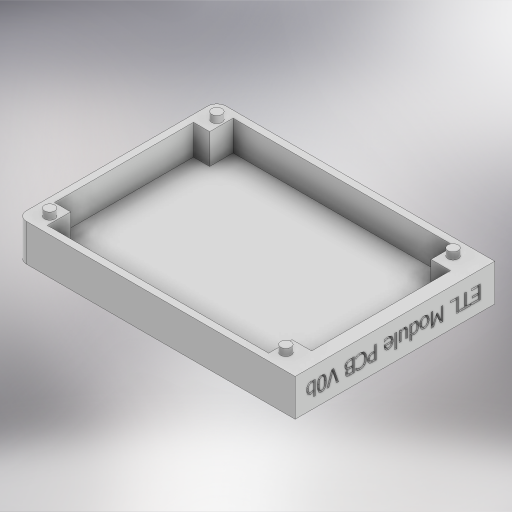
# Autodesk Inventor part: Cover V1
Saved by Autodesk Inventor 2024 (Build 280153000, 153)
## iProperties
Created: 2023-10-11
Part Number: Cover V1
Material: Generic
Document SubType Name: Modeling
Designer: cfang
Density: 1 g/cm^3
Appearance: Default
Author: cfang
Autodesk Inventor part; units mm, degrees
ref_plane "YZ Plane" through (0, 0, 0) normal (1, 0, 0) x (0, 1, 0)
ref_plane "XZ Plane" through (0, 0, 0) normal (0, 1, 0) x (-1, 0, 0)
ref_plane "XY Plane" through (0, 0, 0) normal (0, 0, 1) x (1, 0, 0)
sketch "Sketch1" plane through (0, 0, 0) normal (0, 1, 0) x (-1, 0, 0)
  line L0 (-30, -21.55) -> (30, -21.55)
  line L1 (30, -21.55) -> (30, 21.55)
  line L2 (30, 21.55) -> (-30, 21.55)
  line L3 (-30, 21.55) -> (-30, -21.55)
  line L4 (-30, -21.55) -> (30, 21.55) construction
  line L5 (30, -21.55) -> (-30, 21.55) construction
  point P0 (0, 0)
  dimension "d0" = 43.1
  dimension "d1" = 60
  constraints: 12 end point, 2 midpoint, 2 parallel, 1 horizontal, 1 perpendicular
  measures "d0" distance of L0.end L1.end
  measures "d1" distance of L1.end L2.end
extrude "Extrusion1" add sketch "Sketch1" along normal blind 8
sketch "Sketch2" plane through (0, 8, 0) normal (0, 1, 0) x (1, 0, 0)
  line L0 (22.78, 20.05) -> (-25, 20.05)
  line L1 (-25, 20.05) -> (-25, -20.05)
  line L2 (-25, -20.05) -> (22.78, -20.05)
  line L3 (22.78, -20.05) -> (22.78, 20.05)
  line L4 (-30, -21.55) -> (30, -21.55) projected
  line L5 (30, -21.55) -> (30, 21.55) projected
  line L6 (-30, 21.55) -> (-30, -21.55) projected
  line L7 (30, 21.55) -> (-30, 21.55) projected
  line L8 (22.78, -15) -> (27, -15)
  line L9 (27, -15) -> (27, 15)
  line L10 (27, 15) -> (22.78, 15)
  line L11 (22.78, 15) -> (22.78, -15)
  line L12 (-25, 15) -> (-28.5, 15)
  line L13 (-28.5, 15) -> (-28.5, -15)
  line L14 (-28.5, -15) -> (-25, -15)
  line L15 (-25, -15) -> (-25, 15)
  point P0 (0, 0)
  point P1 (22.78, 15)
  dimension "d4" = 1.5
  dimension "d7" = 7.22
  dimension "d8" = 5
  dimension "d9" = 1.5
  dimension "d24" = 30
  dimension "d25" = 15
  dimension "d26" = 3
  dimension "d27" = 30
  dimension "d28" = 1.5
  dimension "d29" = 15
  constraints: 24 end point, 6 parallel, 3 horizontal, 3 perpendicular, 2 point on line
  measures "d4" distance between parallel lines of L4 L2
  measures "d7" distance between parallel lines of L5 L3
  measures "d8" distance between parallel lines of L6 L1
  measures "d9" distance between parallel lines of L7 L0
  measures "d24" distance of L8.end L9.end
  measures "d25" distance from line of point (0, 0) L10
  measures "d26" distance between parallel lines of L5 L9
  measures "d27" distance of L12.end L13.end
  measures "d28" distance between parallel lines of L6 L13
  measures "d29" distance from line of point (0, 0) L12
extrude "Extrusion2" cut sketch "Sketch2" against normal blind 6.5 contours L3 L2 L1 L0 | L10 L9 L8 L3 | L1 L14 L13 L12
fillet "Fillet1" radius 2 2 edges at (-30, 4, 21.55) (-30, 4, -21.55)
sketch "Sketch3" plane through (0, 8, 0) normal (0, 1, 0) x (1, 0, 0)
  circle A0 centre (24.5, 18.05) radius 1.1
  circle A1 centre (24.5, -18.05) radius 1.1
  line L0 (30, -21.55) -> (30, 21.55) projected
  circle A2 centre (-26.5, 18.05) radius 1.1
  circle A3 centre (-26.5, -18.05) radius 1.1
  line L1 (30, 21.55) -> (-28, 21.55) projected
  point P0 (0, 0)
  dimension "d11" = 2.2
  dimension "d12" = 2.2
  dimension "d13" = 5.5
  dimension "d14" = 2.2
  dimension "d15" = 2.2
  dimension "d16" = 56.5
  dimension "d21" = 36.1
  dimension "d22" = 3.5
  dimension "d23" = 43.1
  constraints: 4 centre point, 2 horizontal alignment, 2 vertical alignment
  measures "d11" diameter of A0
  measures "d12" diameter of A1
  measures "d13" distance from line of L0 A0.centre
  measures "d14" diameter of A2
  measures "d15" diameter of A3
  measures "d16" distance from line of A2.centre L0
  measures "d21" distance of A3.centre A2.centre
  measures "d22" distance from line of L1 A2.centre
  measures "d23" distance of L0.start L0.end
extrude "Extrusion3" add sketch "Sketch3" along normal blind 1.5
sketch "Sketch4" plane through (30, 0, 21.55) normal (1, 0, 0) x (0, 0, -1)
  line L0 (40.589, 2.1906) -> (2.0494, 2.1906) construction
  line L1 (2.0494, 2.1906) -> (2.0494, 11.2351) construction
  line L2 (2.0494, 11.2351) -> (40.589, 11.2351) construction
  line L3 (40.589, 11.2351) -> (40.589, 2.1906) construction
  line L4 (39.9817, 5.3243) -> (39.9817, 2.3243)
  line L5 (39.9817, 2.3243) -> (38.1049, 2.3243)
  line L6 (38.1049, 2.3243) -> (38.1049, 2.6792)
  line L7 (38.1049, 2.6792) -> (39.583, 2.6792)
  line L8 (39.583, 2.6792) -> (39.583, 3.5009)
  line L9 (39.583, 3.5009) -> (38.2046, 3.5009)
  line L10 (38.2046, 3.5009) -> (38.2046, 3.8559)
  line L11 (38.2046, 3.8559) -> (39.583, 3.8559)
  line L12 (39.583, 3.8559) -> (39.583, 4.9693)
  line L13 (39.583, 4.9693) -> (38.1049, 4.9693)
  line L14 (38.1049, 4.9693) -> (38.1049, 5.3243)
  line L15 (38.1049, 5.3243) -> (39.9817, 5.3243)
  line L16 (36.9671, 5.3243) -> (36.9671, 2.6792)
  line L17 (36.9671, 2.6792) -> (37.9736, 2.6792)
  line L18 (37.9736, 2.6792) -> (37.9736, 2.3243)
  line L19 (37.9736, 2.3243) -> (35.5619, 2.3243)
  line L20 (35.5619, 2.3243) -> (35.5619, 2.6792)
  line L21 (35.5619, 2.6792) -> (36.5684, 2.6792)
  line L22 (36.5684, 2.6792) -> (36.5684, 5.3243)
  line L23 (36.5684, 5.3243) -> (36.9671, 5.3243)
  line L24 (33.5198, 5.3243) -> (35.258, 5.3243)
  line L25 (35.258, 5.3243) -> (35.258, 2.3243)
  line L26 (35.258, 2.3243) -> (34.8593, 2.3243)
  line L27 (34.8593, 2.3243) -> (34.8593, 4.9693)
  line L28 (34.8593, 4.9693) -> (33.5198, 4.9693)
  line L29 (33.5198, 4.9693) -> (33.5198, 5.3243)
  line L30 (29.3456, 5.3243) -> (29.7443, 5.3243)
  line L31 (29.7443, 5.3243) -> (29.7443, 2.74)
  line L32 (29.7443, 2.74) -> (30.5271, 4.4977)
  line L33 (30.5271, 4.4977) -> (30.7702, 4.4977)
  line L34 (30.7702, 4.4977) -> (31.5457, 2.74)
  line L35 (31.5457, 2.74) -> (31.5457, 5.3243)
  line L36 (31.5457, 5.3243) -> (31.9177, 5.3243)
  line L37 (31.9177, 5.3243) -> (31.9177, 2.3243)
  line L38 (31.9177, 2.3243) -> (31.3731, 2.3243)
  line L39 (31.3731, 2.3243) -> (30.6243, 3.9944)
  line L40 (30.6243, 3.9944) -> (29.8999, 2.3243)
  line L41 (29.8999, 2.3243) -> (29.3456, 2.3243)
  line L42 (29.3456, 2.3243) -> (29.3456, 5.3243)
  spline S0 degree 2 poles (26.9169, 4.1987) (26.9169, 4.7675) (27.4639, 5.3875) (27.9209, 5.3875) knots 0 0 0 1 2 2 2
  spline S1 degree 2 poles (27.9209, 5.3875) (28.3901, 5.3875) (28.9274, 4.7481) (28.9274, 4.1987) knots 0 0 0 1 2 2 2
  spline S2 degree 2 poles (28.9274, 4.1987) (28.9274, 3.6346) (28.3731, 3.0098) (27.9209, 3.0098) knots 0 0 0 1 2 2 2
  spline S3 degree 2 poles (27.9209, 3.0098) (27.4639, 3.0098) (26.9169, 3.6322) (26.9169, 4.1987) knots 0 0 0 1 2 2 2
  spline S4 degree 2 poles (27.3083, 4.1987) (27.3083, 3.7611) (27.6268, 3.3356) (27.9209, 3.3356) knots 0 0 0 1 2 2 2
  spline S5 degree 2 poles (27.9209, 3.3356) (28.2151, 3.3356) (28.536, 3.7611) (28.536, 4.1987) knots 0 0 0 1 2 2 2
  spline S6 degree 2 poles (28.536, 4.1987) (28.536, 4.6241) (28.2151, 5.0617) (27.9209, 5.0617) knots 0 0 0 1 2 2 2
  spline S7 degree 2 poles (27.9209, 5.0617) (27.6292, 5.0617) (27.3083, 4.6314) (27.3083, 4.1987) knots 0 0 0 1 2 2 2
  line L43 (24.7969, 5.3243) -> (25.1762, 5.3243)
  line L44 (25.1762, 5.3243) -> (25.1762, 5.0957)
  spline S8 degree 2 poles (25.1762, 5.0957) (25.2637, 5.1687) (25.3926, 5.2659) (25.4801, 5.3072) knots 0 0 0 1 2 2 2
  spline S9 degree 2 poles (25.4801, 5.3072) (25.5603, 5.3461) (25.7329, 5.3875) (25.8472, 5.3875) knots 0 0 0 1 2 2 2
  spline S10 degree 2 poles (25.8472, 5.3875) (26.0319, 5.3875) (26.3431, 5.2343) (26.4525, 5.086) knots 0 0 0 1 2 2 2
  spline S11 degree 2 poles (26.4525, 5.086) (26.5619, 4.9377) (26.6835, 4.5001) (26.6835, 4.2157) knots 0 0 0 1 2 2 2
  spline S12 degree 2 poles (26.6835, 4.2157) (26.6835, 3.9191) (26.5303, 3.4863) (26.3966, 3.3235) knots 0 0 0 1 2 2 2
  spline S13 degree 2 poles (26.3966, 3.3235) (26.2726, 3.1776) (25.925, 3.0098) (25.7329, 3.0098) knots 0 0 0 1 2 2 2
  spline S14 degree 2 poles (25.7329, 3.0098) (25.5652, 3.0098) (25.3148, 3.0852) (25.1762, 3.163) knots 0 0 0 1 2 2 2
  line L45 (25.1762, 3.163) -> (25.1762, 2.1906)
  line L46 (25.1762, 2.1906) -> (24.7969, 2.1906)
  line L47 (24.7969, 2.1906) -> (24.7969, 5.3243)
  line L48 (25.1762, 4.7773) -> (25.1762, 3.4766)
  spline S15 degree 2 poles (25.1762, 3.4766) (25.3172, 3.4085) (25.5409, 3.3575) (25.6697, 3.3575) knots 0 0 0 1 2 2 2
  spline S16 degree 2 poles (25.6697, 3.3575) (25.9614, 3.3575) (26.2921, 3.7951) (26.2921, 4.2084) knots 0 0 0 1 2 2 2
  spline S17 degree 2 poles (26.2921, 4.2084) (26.2921, 4.6071) (26.0392, 5.0277) (25.7597, 5.0277) knots 0 0 0 1 2 2 2
  spline S18 degree 2 poles (25.7597, 5.0277) (25.6114, 5.0277) (25.3099, 4.8915) (25.1762, 4.7773) knots 0 0 0 1 2 2 2
  line L49 (22.4971, 5.3243) -> (22.8764, 5.3243)
  line L50 (22.8764, 5.3243) -> (22.8764, 5.0763)
  spline S19 degree 2 poles (22.8764, 5.0763) (23.0514, 5.2295) (23.365, 5.3875) (23.5595, 5.3875) knots 0 0 0 1 2 2 2
  spline S20 degree 2 poles (23.5595, 5.3875) (23.7054, 5.3875) (23.9655, 5.2902) (24.0603, 5.1857) knots 0 0 0 1 2 2 2
  spline S21 degree 2 poles (24.0603, 5.1857) (24.1575, 5.0812) (24.2645, 4.7627) (24.2645, 4.5342) knots 0 0 0 1 2 2 2
  line L51 (24.2645, 4.5342) -> (24.2645, 3.0731)
  line L52 (24.2645, 3.0731) -> (23.8853, 3.0731)
  line L53 (23.8853, 3.0731) -> (23.8853, 4.3567)
  spline S22 degree 2 poles (23.8853, 4.3567) (23.8853, 4.5366) (23.8585, 4.7724) (23.8123, 4.8599) knots 0 0 0 1 2 2 2
  spline S23 degree 2 poles (23.8123, 4.8599) (23.7661, 4.9474) (23.6081, 5.0277) (23.4598, 5.0277) knots 0 0 0 1 2 2 2
  spline S24 degree 2 poles (23.4598, 5.0277) (23.3212, 5.0277) (23.0076, 4.8696) (22.8764, 4.7554) knots 0 0 0 1 2 2 2
  line L54 (22.8764, 4.7554) -> (22.8764, 3.0731)
  line L55 (22.8764, 3.0731) -> (22.4971, 3.0731)
  line L56 (22.4971, 3.0731) -> (22.4971, 5.3243)
  line L57 (21.5611, 5.3243) -> (21.9404, 5.3243)
  line L58 (21.9404, 5.3243) -> (21.9404, 2.1906)
  line L59 (21.9404, 2.1906) -> (21.5611, 2.1906)
  line L60 (21.5611, 2.1906) -> (21.5611, 5.3243)
  spline S25 degree 2 poles (20.0271, 5.3753) (20.5668, 5.3753) (21.16, 4.77) (21.16, 4.2108) knots 0 0 0 1 2 2 2
  spline S26 degree 2 poles (21.16, 4.2108) (21.16, 3.6614) (20.5838, 3.0098) (20.1195, 3.0098) knots 0 0 0 1 2 2 2
  spline S27 degree 2 poles (20.1195, 3.0098) (19.9104, 3.0098) (19.587, 3.1314) (19.4679, 3.2602) knots 0 0 0 1 2 2 2
  spline S28 degree 2 poles (19.4679, 3.2602) (19.3464, 3.3891) (19.2175, 3.7611) (19.2175, 4.0309) knots 0 0 0 1 2 2 2
  line L61 (19.2175, 4.0309) -> (19.2175, 4.2376)
  line L62 (19.2175, 4.2376) -> (20.7759, 4.2376)
  spline S29 degree 2 poles (20.7759, 4.2376) (20.7759, 4.629) (20.382, 5.0447) (20.0319, 5.0447) knots 0 0 0 1 2 2 2
  spline S30 degree 2 poles (20.0319, 5.0447) (19.908, 5.0447) (19.6673, 4.9888) (19.57, 4.945) knots 0 0 0 1 2 2 2
  spline S31 degree 2 poles (19.57, 4.945) (19.4679, 4.8964) (19.3269, 4.8113) (19.2807, 4.7724) knots 0 0 0 1 2 2 2
  line L63 (19.2807, 4.7724) -> (19.2588, 4.7724)
  line L64 (19.2588, 4.7724) -> (19.2588, 5.1857)
  spline S32 degree 2 poles (19.2588, 5.1857) (19.3245, 5.2124) (19.5238, 5.2902) (19.6016, 5.3121) knots 0 0 0 1 2 2 2
  spline S33 degree 2 poles (19.6016, 5.3121) (19.711, 5.3437) (19.8909, 5.3753) (20.0271, 5.3753) knots 0 0 0 1 2 2 2
  spline S34 degree 2 poles (19.587, 3.9483) (19.5919, 3.7951) (19.6551, 3.5714) (19.7159, 3.4961) knots 0 0 0 1 2 2 2
  spline S35 degree 2 poles (19.7159, 3.4961) (19.7815, 3.411) (19.9882, 3.321) (20.1413, 3.321) knots 0 0 0 1 2 2 2
  spline S36 degree 2 poles (20.1413, 3.321) (20.2921, 3.321) (20.5036, 3.411) (20.5911, 3.4985) knots 0 0 0 1 2 2 2
  spline S37 degree 2 poles (20.5911, 3.4985) (20.6762, 3.5884) (20.7637, 3.8048) (20.7759, 3.9483) knots 0 0 0 1 2 2 2
  line L65 (20.7759, 3.9483) -> (19.587, 3.9483)
  spline S38 degree 2 poles (15.6195, 3.2286) (15.6195, 3.4231) (15.758, 3.7732) (15.882, 3.8948) knots 0 0 0 1 2 2 2
  spline S39 degree 2 poles (15.882, 3.8948) (16.0376, 4.0479) (16.4582, 4.206) (16.7791, 4.206) knots 0 0 0 1 2 2 2
  line L66 (16.7791, 4.206) -> (17.117, 4.206)
  line L67 (17.117, 4.206) -> (17.117, 5.3243)
  line L68 (17.117, 5.3243) -> (17.5157, 5.3243)
  line L69 (17.5157, 5.3243) -> (17.5157, 2.3243)
  line L70 (17.5157, 2.3243) -> (16.7621, 2.3243)
  spline S40 degree 2 poles (16.7621, 2.3243) (16.4947, 2.3243) (16.1203, 2.4118) (15.9768, 2.5115) knots 0 0 0 1 2 2 2
  spline S41 degree 2 poles (15.9768, 2.5115) (15.8091, 2.6257) (15.6195, 2.9782) (15.6195, 3.2286) knots 0 0 0 1 2 2 2
  spline S42 degree 2 poles (16.0352, 3.2408) (16.0352, 3.0852) (16.1422, 2.8567) (16.2516, 2.7837) knots 0 0 0 1 2 2 2
  spline S43 degree 2 poles (16.2516, 2.7837) (16.3464, 2.7205) (16.5992, 2.6695) (16.7864, 2.6695) knots 0 0 0 1 2 2 2
  line L71 (16.7864, 2.6695) -> (17.117, 2.6695)
  line L72 (17.117, 2.6695) -> (17.117, 3.8656)
  line L73 (17.117, 3.8656) -> (16.8447, 3.8656)
  spline S44 degree 2 poles (16.8447, 3.8656) (16.6016, 3.8656) (16.3026, 3.7878) (16.2054, 3.6857) knots 0 0 0 1 2 2 2
  spline S45 degree 2 poles (16.2054, 3.6857) (16.1154, 3.5957) (16.0352, 3.3842) (16.0352, 3.2408) knots 0 0 0 1 2 2 2
  spline S46 degree 2 poles (14.0684, 5.3778) (14.3601, 5.3778) (14.8537, 5.1808) (15.0336, 4.9839) knots 0 0 0 1 2 2 2
  spline S47 degree 2 poles (15.0336, 4.9839) (15.2135, 4.7894) (15.4104, 4.206) (15.4104, 3.8267) knots 0 0 0 1 2 2 2
  spline S48 degree 2 poles (15.4104, 3.8267) (15.4104, 3.4499) (15.2183, 2.8907) (15.036, 2.6841) knots 0 0 0 1 2 2 2
  spline S49 degree 2 poles (15.036, 2.6841) (14.8561, 2.4823) (14.365, 2.2708) (14.0611, 2.2708) knots 0 0 0 1 2 2 2
  spline S50 degree 2 poles (14.0611, 2.2708) (13.9104, 2.2708) (13.6454, 2.3145) (13.5336, 2.3486) knots 0 0 0 1 2 2 2
  spline S51 degree 2 poles (13.5336, 2.3486) (13.4363, 2.3802) (13.2345, 2.4701) (13.1349, 2.5236) knots 0 0 0 1 2 2 2
  line L74 (13.1349, 2.5236) -> (13.1349, 3.005)
  line L75 (13.1349, 3.005) -> (13.1665, 3.005)
  spline S52 degree 2 poles (13.1665, 3.005) (13.2199, 2.9564) (13.3853, 2.8202) (13.5044, 2.7546) knots 0 0 0 1 2 2 2
  spline S53 degree 2 poles (13.5044, 2.7546) (13.6187, 2.6914) (13.8885, 2.6111) (14.0635, 2.6111) knots 0 0 0 1 2 2 2
  spline S54 degree 2 poles (14.0635, 2.6111) (14.2556, 2.6111) (14.5984, 2.7692) (14.7272, 2.9199) knots 0 0 0 1 2 2 2
  spline S55 degree 2 poles (14.7272, 2.9199) (14.8537, 3.0731) (14.9947, 3.5374) (14.9947, 3.8267) knots 0 0 0 1 2 2 2
  spline S56 degree 2 poles (14.9947, 3.8267) (14.9947, 4.1354) (14.8464, 4.5803) (14.7175, 4.7335) knots 0 0 0 1 2 2 2
  spline S57 degree 2 poles (14.7175, 4.7335) (14.5911, 4.8818) (14.2532, 5.0325) (14.0635, 5.0325) knots 0 0 0 1 2 2 2
  spline S58 degree 2 poles (14.0635, 5.0325) (13.8909, 5.0325) (13.5968, 4.9474) (13.4825, 4.8842) knots 0 0 0 1 2 2 2
  spline S59 degree 2 poles (13.4825, 4.8842) (13.3731, 4.821) (13.2102, 4.6897) (13.164, 4.6436) knots 0 0 0 1 2 2 2
  line L76 (13.164, 4.6436) -> (13.1349, 4.6436)
  line L77 (13.1349, 4.6436) -> (13.1349, 5.1201)
  spline S60 degree 2 poles (13.1349, 5.1201) (13.2345, 5.1662) (13.4096, 5.2513) (13.5336, 5.2902) knots 0 0 0 1 2 2 2
  spline S61 degree 2 poles (13.5336, 5.2902) (13.6648, 5.334) (13.8885, 5.3778) (14.0684, 5.3778) knots 0 0 0 1 2 2 2
  spline S62 degree 2 poles (10.7281, 4.4029) (10.7281, 4.6265) (10.8982, 4.9693) (11.0392, 5.0812) knots 0 0 0 1 2 2 2
  spline S63 degree 2 poles (11.0392, 5.0812) (11.2094, 5.2124) (11.596, 5.3243) (11.9023, 5.3243) knots 0 0 0 1 2 2 2
  line L78 (11.9023, 5.3243) -> (12.7629, 5.3243)
  line L79 (12.7629, 5.3243) -> (12.7629, 2.3243)
  line L80 (12.7629, 2.3243) -> (11.9679, 2.3243)
  spline S64 degree 2 poles (11.9679, 2.3243) (11.647, 2.3243) (11.3261, 2.3656) (11.1802, 2.4458) knots 0 0 0 1 2 2 2
  spline S65 degree 2 poles (11.1802, 2.4458) (11.0174, 2.5309) (10.8691, 2.8105) (10.8691, 3.0001) knots 0 0 0 1 2 2 2
  spline S66 degree 2 poles (10.8691, 3.0001) (10.8691, 3.2116) (11.0927, 3.5471) (11.2896, 3.6419) knots 0 0 0 1 2 2 2
  line L81 (11.2896, 3.6419) -> (11.2896, 3.6565)
  spline S67 degree 2 poles (11.2896, 3.6565) (11.0222, 3.7295) (10.7281, 4.116) (10.7281, 4.4029) knots 0 0 0 1 2 2 2
  spline S68 degree 2 poles (11.1438, 4.4199) (11.1438, 4.2497) (11.241, 4.0309) (11.3869, 3.9531) knots 0 0 0 1 2 2 2
  spline S69 degree 2 poles (11.3869, 3.9531) (11.4817, 3.9045) (11.7054, 3.8753) (11.912, 3.8753) knots 0 0 0 1 2 2 2
  line L82 (11.912, 3.8753) -> (12.3642, 3.8753)
  line L83 (12.3642, 3.8753) -> (12.3642, 4.9839)
  line L84 (12.3642, 4.9839) -> (12.0409, 4.9839)
  spline S70 degree 2 poles (12.0409, 4.9839) (11.7783, 4.9839) (11.4768, 4.9353) (11.3601, 4.8575) knots 0 0 0 1 2 2 2
  spline S71 degree 2 poles (11.3601, 4.8575) (11.2483, 4.7773) (11.1438, 4.5779) (11.1438, 4.4199) knots 0 0 0 1 2 2 2
  spline S72 degree 2 poles (11.2848, 3.056) (11.2848, 2.9491) (11.3577, 2.7886) (11.4379, 2.7424) knots 0 0 0 1 2 2 2
  spline S73 degree 2 poles (11.4379, 2.7424) (11.5352, 2.6889) (11.771, 2.6646) (11.9825, 2.6646) knots 0 0 0 1 2 2 2
  line L85 (11.9825, 2.6646) -> (12.3642, 2.6646)
  line L86 (12.3642, 2.6646) -> (12.3642, 3.5423)
  line L87 (12.3642, 3.5423) -> (11.912, 3.5423)
  spline S74 degree 2 poles (11.912, 3.5423) (11.7248, 3.5423) (11.5473, 3.5034) (11.4525, 3.4426) knots 0 0 0 1 2 2 2
  spline S75 degree 2 poles (11.4525, 3.4426) (11.3601, 3.3842) (11.2848, 3.197) (11.2848, 3.056) knots 0 0 0 1 2 2 2
  line L88 (6.8674, 2.3243) -> (7.9007, 5.3243)
  line L89 (7.9007, 5.3243) -> (8.331, 5.3243)
  line L90 (8.331, 5.3243) -> (9.3642, 2.3243)
  line L91 (9.3642, 2.3243) -> (8.9363, 2.3243)
  line L92 (8.9363, 2.3243) -> (8.1049, 4.8162)
  line L93 (8.1049, 4.8162) -> (7.2734, 2.3243)
  line L94 (7.2734, 2.3243) -> (6.8674, 2.3243)
  spline S76 degree 2 poles (4.7986, 3.8243) (4.7986, 4.6314) (5.2678, 5.3875) (5.7564, 5.3875) knots 0 0 0 1 2 2 2
  spline S77 degree 2 poles (5.7564, 5.3875) (6.2524, 5.3875) (6.7167, 4.6168) (6.7167, 3.8267) knots 0 0 0 1 2 2 2
  spline S78 degree 2 poles (6.7167, 3.8267) (6.7167, 3.0147) (6.2475, 2.2635) (5.7564, 2.2635) knots 0 0 0 1 2 2 2
  spline S79 degree 2 poles (5.7564, 2.2635) (5.2629, 2.2635) (4.7986, 3.0414) (4.7986, 3.8243) knots 0 0 0 1 2 2 2
  spline S80 degree 2 poles (5.314, 4.7384) (5.2556, 4.5901) (5.207, 4.133) (5.207, 3.8243) knots 0 0 0 1 2 2 2
  spline S81 degree 2 poles (5.207, 3.8243) (5.207, 3.5155) (5.2556, 3.0609) (5.3164, 2.9077) knots 0 0 0 1 2 2 2
  spline S82 degree 2 poles (5.3164, 2.9077) (5.3772, 2.7546) (5.5887, 2.5966) (5.7564, 2.5966) knots 0 0 0 1 2 2 2
  spline S83 degree 2 poles (5.7564, 2.5966) (5.9242, 2.5966) (6.1405, 2.7546) (6.2037, 2.9126) knots 0 0 0 1 2 2 2
  spline S84 degree 2 poles (6.2037, 2.9126) (6.2645, 3.0658) (6.3083, 3.5325) (6.3083, 3.8267) knots 0 0 0 1 2 2 2
  spline S85 degree 2 poles (6.3083, 3.8267) (6.3083, 4.1427) (6.2694, 4.5658) (6.2062, 4.7311) knots 0 0 0 1 2 2 2
  spline S86 degree 2 poles (6.2062, 4.7311) (6.1478, 4.8867) (5.9315, 5.0544) (5.7564, 5.0544) knots 0 0 0 1 2 2 2
  spline S87 degree 2 poles (5.7564, 5.0544) (5.5911, 5.0544) (5.3747, 4.8964) (5.314, 4.7384) knots 0 0 0 1 2 2 2
  spline S88 degree 2 poles (2.472, 4.1622) (2.472, 4.7141) (3.0068, 5.3875) (3.4104, 5.3875) knots 0 0 0 1 2 2 2
  spline S89 degree 2 poles (3.4104, 5.3875) (3.5927, 5.3875) (3.8528, 5.2975) (3.9793, 5.2197) knots 0 0 0 1 2 2 2
  line L95 (3.9793, 5.2197) -> (4.0036, 5.3243)
  line L96 (4.0036, 5.3243) -> (4.3585, 5.3243)
  line L97 (4.3585, 5.3243) -> (4.3585, 2.1906)
  line L98 (4.3585, 2.1906) -> (3.9793, 2.1906)
  line L99 (3.9793, 2.1906) -> (3.9793, 3.3089)
  spline S90 degree 2 poles (3.9793, 3.3089) (3.8358, 3.18) (3.5028, 3.0098) (3.2913, 3.0098) knots 0 0 0 1 2 2 2
  spline S91 degree 2 poles (3.2913, 3.0098) (2.9096, 3.0098) (2.472, 3.6201) (2.472, 4.1622) knots 0 0 0 1 2 2 2
  spline S92 degree 2 poles (2.8634, 4.1914) (2.8634, 3.7878) (3.1089, 3.3696) (3.3812, 3.3696) knots 0 0 0 1 2 2 2
  spline S93 degree 2 poles (3.3812, 3.3696) (3.5344, 3.3696) (3.8504, 3.5155) (3.9793, 3.6273) knots 0 0 0 1 2 2 2
  line L100 (3.9793, 3.6273) -> (3.9793, 4.9183)
  spline S94 degree 2 poles (3.9793, 4.9183) (3.8358, 4.9888) (3.6146, 5.0471) (3.4833, 5.0471) knots 0 0 0 1 2 2 2
  spline S95 degree 2 poles (3.4833, 5.0471) (3.194, 5.0471) (2.8634, 4.6363) (2.8634, 4.1914) knots 0 0 0 1 2 2 2
  point P0 (21.55, 0)
  constraints: 2 other
emboss "Emboss1" sketch "Sketch4" operation cut depth 1 direction (-1, 0, 0)
equation "\"d9\" = d4"
equation "\"d25\" = 0.5 * d24"
equation "\"d27\" = d24"
equation "\"d29\" = d25"
equation "\"d12\" = d11"
equation "\"d14\" = d11"
equation "\"d15\" = d11"
equation "\"d22\" = -0.5 * d21 + 0.5 * d23"
body "Solid1"
